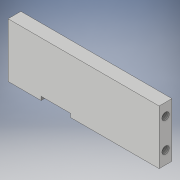
# Autodesk Inventor part: USB Wärmeableiter 1
Saved by Autodesk Inventor 2017 (Build 210142000, 142)
## iProperties
Part Number: USB Wärmeableiter 1
Material: Generisch
Document SubType Name: Modeling
Designer: David Merges
Density: 1 g/cm^3
Appearance: Vorgabe
Author: David Merges
Autodesk Inventor part; units mm, degrees
ref_plane "YZ Plane" through (0, 0, 0) normal (1, 0, 0) x (0, 1, 0)
ref_plane "XZ Plane" through (0, 0, 0) normal (0, 1, 0) x (-1, 0, 0)
sketch "Skizze1" plane through (0, 0, 0) normal (0, 0, 1) x (1, 0, 0)
  line L0 (0, 1.75) -> (41.2, 1.75)
  line L1 (41.2, 1.75) -> (41.2, -1.75)
  line L2 (41.2, -1.75) -> (0, -1.75)
  line L3 (0, -1.75) -> (0, 1.75)
  point P0 (0, 0)
  point P1 (0, 0)
  dimension "d0" = 41.2
  dimension "d1" = 3.5
  constraints: 8 end point, 2 parallel, 1 coincident, 1 horizontal, 1 midpoint, 1 perpendicular
  measures "d0" distance of L0.start L0.end
  measures "d1" distance of L2.end L0.start
extrude "Extrusion1" add sketch "Skizze1" along normal blind 14.8
sketch "Skizze2" plane through (0, 0, 0) normal (0, 0, -1) x (-1, 0, 0)
  line L0 (0, 0) -> (-3, 0) construction
  line L1 (-3, 0) -> (-32, 0) construction
  dimension "d4" = 3
  dimension "d5" = 32
  constraints: 4 end point, 2 coincident, 1 horizontal, 1 point on line
  measures "d4" distance of L0.start L0.end
  measures "d5" distance of L0.start L1.end
hole "Bohrung1" at (3, 0, 0) at (32, 0, 0) direction (0, 0, 1) diameter 2.013 depth 9 tip angle 118 thread size "M2.5x0.45" class "6H" standard "ISO Metric profile"
sketch "Skizze3" plane through (0, 0, 0) normal (0, 0, -1) x (-1, 0, 0)
  circle A0 centre (-3, 0) radius 1.0065 projected
  circle A1 centre (-32, 0) radius 1.0065 projected
  line L0 (0, 1.75) -> (-41.2, 1.75) projected
  line L1 (-41.2, 1.75) -> (-41.2, -1.75) projected
  line L2 (-41.2, -1.75) -> (0, -1.75) projected
  line L3 (0, -1.75) -> (0, 1.75) projected
  line L4 (-41.2, -1.75) -> (0, -1.75) projected
  line L5 (-9, -1.75) -> (-17, -1.75)
  line L6 (-17, -1.75) -> (-17, 1.75)
  line L7 (-17, 1.75) -> (-9, 1.75)
  line L8 (-9, 1.75) -> (-9, -1.75)
  line L9 (-17, 0) -> (-9, 0) construction
  point P0 (0, 0)
  point P1 (-13, 0)
  dimension "d13" = 13
  dimension "d14" = 8
  constraints: 10 end point, 3 midpoint, 2 parallel, 2 point on line, 1 horizontal, 1 perpendicular
  measures "d13" distance from line of L3 point (-13, 0)
  measures "d14" distance between parallel lines of L6 L8
extrude "Extrusion2" cut sketch "Skizze3" against normal blind 1 contours L8 L2 L6 L0
sketch "Skizze4" plane through (41.2, -1.75, 0) normal (1, 0, 0) x (0, 0, -1)
  line L0 (0, 1.75) -> (-3.5, 1.75) construction
  line L1 (-3.5, 1.75) -> (-11.5, 1.75) construction
  dimension "d17" = 3.5
  dimension "d19" = 8
  constraints: 4 end point, 1 horizontal, 1 point on line
  measures "d17" distance of L0.start L0.end
  measures "d19" distance of L0.end L1.end
hole "Bohrung2" at (41.2, 0, 11.5) at (41.2, 0, 3.5) direction (-1, 0, 0) diameter 2.013 depth 7 tip angle 118 thread size "M2.5x0.45" class "6H" standard "ISO Metric profile"
ref_plane "Arbeitsebene1" through (0, 0, 7.4) normal (0, 0, 1) x (1, 0, 0)
